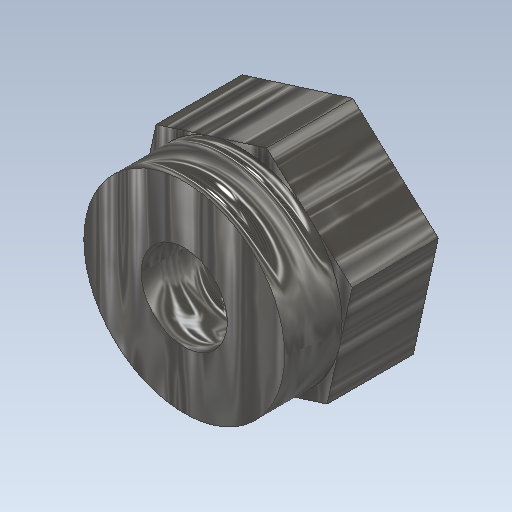
# Autodesk Inventor part: ナイロンナットm4
Saved by Autodesk Inventor 2020.2 (Build 242310000, 310)
## iProperties
Created: 2016-02-22
Part Number: ナイロンナットm4
Material: ステンレス鋼
Document SubType Name: Modeling
Designer: Takumi
Density: 8 g/cm^3
Appearance: つや出し ブラシ仕上げ
Mass: 1.35145 g
Surface Area: 2.34586 cm^2
Volume: 0.168932 cm^3
Author: Takumi
Autodesk Inventor part; units mm, degrees
ref_plane "YZ Plane" through (0, 0, 0) normal (1, 0, 0) x (0, 1, 0)
ref_plane "XZ Plane" through (0, 0, 0) normal (0, 1, 0) x (-1, 0, 0)
ref_plane "XY Plane" through (0, 0, 0) normal (0, 0, 1) x (1, 0, 0)
sketch "スケッチ1" plane through (0, 0, 0) normal (0, 0, 1) x (1, 0, 0)
  line L0 (3.8535, 1.2181) -> (2.9816, -2.7282)
  line L1 (2.9816, -2.7282) -> (-0.8719, -3.9463)
  line L2 (-0.8719, -3.9463) -> (-3.8535, -1.2181)
  line L3 (-3.8535, -1.2181) -> (-2.9816, 2.7282)
  line L4 (-2.9816, 2.7282) -> (0.8719, 3.9463)
  line L5 (0.8719, 3.9463) -> (3.8535, 1.2181)
  circle A0 centre (0, 0) radius 3.5
  dimension "d0" = 8.0829
  dimension "d1" = 7
  constraints: 12 end point, 2 coincident, 1 centre point, 1 tangent, 13 other
  measures "d0" distance of L4.end L1.end
  measures "d1" distance of L0.end L2.end
extrude "押し出し1" add sketch "スケッチ1" along normal blind 2 contours A0
extrude "押し出し2" add sketch "スケッチ1" against normal blind 3
hole "穴1" at (0, 0, 0) direction (0, 0, -1) diameter 3 end through all
hole "穴2" at (0, 0, 0) direction (0, 0, 1) diameter 3 end through all
